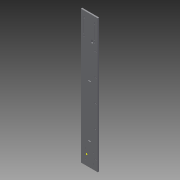
# Autodesk Inventor part: Tenda Wifi Buoy Mounting Plate
Saved by Autodesk Inventor 2015 (Build 190159000, 159)
## iProperties
Created: 2015-07-10
Part Number: Tenda Wifi Buoy Mounting Plate
Material: Generic
Document SubType Name: Modeling
Designer: Carey
Density: 1 g/cm^3
Appearance: Default
Author: Carey
Autodesk Inventor part; units mm, degrees
ref_plane "YZ Plane" through (0, 0, 0) normal (1, 0, 0) x (0, 1, 0)
ref_plane "XZ Plane" through (0, 0, 0) normal (0, 1, 0) x (-1, 0, 0)
ref_plane "XY Plane" through (0, 0, 0) normal (0, 0, 1) x (1, 0, 0)
sketch "Sketch1" plane through (0, 0, 0) normal (0, 0, 1) x (1, 0, 0)
  point P0 (0, 0)
sketch "Sketch2" plane through (0, 0, 0) normal (0, 0, 1) x (1, 0, 0)
  line L0 (-26.773, -46.7791) -> (49.427, -46.7791)
  line L1 (49.427, -46.7791) -> (49.427, 556.4709)
  line L2 (-26.773, 556.4709) -> (-26.773, -46.7791)
  line L3 (-13.7555, 533.9284) -> (-11.8505, 533.9284)
  line L4 (-11.8505, 533.9284) -> (-11.8505, 525.9909)
  line L5 (-11.8505, 525.9909) -> (-13.7555, 525.9909)
  line L6 (-13.7555, 525.9909) -> (-13.7555, 533.9284)
  line L7 (46.252, 424.6449) -> (44.347, 424.6449)
  line L8 (44.347, 424.6449) -> (44.347, 419.5649)
  line L9 (44.347, 419.5649) -> (46.252, 419.5649)
  line L10 (46.252, 419.5649) -> (46.252, 424.6449)
  line L11 (36.5111, 522.1809) -> (36.5111, 463.7609)
  line L12 (36.5111, 463.7609) -> (35.457, 463.7609)
  line L13 (35.457, 463.7609) -> (35.457, 522.1809)
  line L14 (35.457, 522.1809) -> (36.5111, 522.1809)
  line L15 (-13.7555, 522.1809) -> (-13.7555, 463.7609)
  line L16 (-13.7555, 463.7609) -> (-12.7014, 463.7609)
  line L17 (-12.7014, 463.7609) -> (-12.7014, 522.1809)
  line L18 (-12.7014, 522.1809) -> (-13.7555, 522.1809)
  line L19 (26.8845, 445.2941) -> (18.947, 445.2941)
  line L20 (18.947, 445.2941) -> (18.947, 457.9824)
  line L21 (18.947, 457.9824) -> (26.8845, 457.9824)
  line L22 (26.8845, 457.9824) -> (26.8845, 445.2941)
  line L23 (11.327, 54.8209) -> (17.677, 54.8209)
  line L24 (17.677, 54.8209) -> (17.677, 58.3769)
  line L25 (17.677, 58.3769) -> (4.977, 58.3769)
  line L26 (4.977, 58.3769) -> (4.977, 54.8209)
  line L27 (4.977, 54.8209) -> (11.327, 54.8209)
  line L28 (11.327, 293.7079) -> (17.677, 293.7079)
  line L29 (17.677, 293.7079) -> (17.677, 290.1519)
  line L30 (17.677, 290.1519) -> (4.977, 290.1519)
  line L31 (4.977, 290.1519) -> (4.977, 293.7079)
  line L32 (4.977, 293.7079) -> (11.327, 293.7079)
  line L33 (36.092, 424.6449) -> (37.997, 424.6449)
  line L34 (37.997, 424.6449) -> (37.997, 419.5649)
  line L35 (37.997, 419.5649) -> (36.092, 419.5649)
  line L36 (36.092, 419.5649) -> (36.092, 424.6449)
  line L37 (46.252, 323.0449) -> (44.347, 323.0449)
  line L38 (44.347, 323.0449) -> (44.347, 317.9649)
  line L39 (44.347, 317.9649) -> (46.252, 317.9649)
  line L40 (46.252, 317.9649) -> (46.252, 323.0449)
  line L41 (36.092, 323.0449) -> (37.997, 323.0449)
  line L42 (37.997, 323.0449) -> (37.997, 317.9649)
  line L43 (37.997, 317.9649) -> (36.092, 317.9649)
  line L44 (36.092, 317.9649) -> (36.092, 323.0449)
  line L45 (46.252, 221.4449) -> (44.347, 221.4449)
  line L46 (44.347, 221.4449) -> (44.347, 216.3649)
  line L47 (44.347, 216.3649) -> (46.252, 216.3649)
  line L48 (46.252, 216.3649) -> (46.252, 221.4449)
  line L49 (36.092, 221.4449) -> (37.997, 221.4449)
  line L50 (37.997, 221.4449) -> (37.997, 216.3649)
  line L51 (37.997, 216.3649) -> (36.092, 216.3649)
  line L52 (36.092, 216.3649) -> (36.092, 221.4449)
  line L53 (46.252, 0.1368) -> (44.347, 0.1368)
  line L54 (44.347, 0.1368) -> (44.347, -4.9432)
  line L55 (44.347, -4.9432) -> (46.252, -4.9432)
  line L56 (46.252, -4.9432) -> (46.252, 0.1368)
  line L57 (36.092, 0.1368) -> (37.997, 0.1368)
  line L58 (37.997, 0.1368) -> (37.997, -4.9432)
  line L59 (37.997, -4.9432) -> (36.092, -4.9432)
  line L60 (36.092, -4.9432) -> (36.092, 0.1368)
  line L61 (49.427, 556.4709) -> (-26.773, 556.4709)
  line L62 (46.252, 424.6449) -> (147.852, 424.6449) construction
  line L63 (46.252, 119.8449) -> (147.852, 119.8449) construction
  line L64 (46.252, 119.8449) -> (44.347, 119.8449)
  line L65 (44.347, 119.8449) -> (44.347, 114.7649)
  line L66 (44.347, 114.7649) -> (46.252, 114.7649)
  line L67 (46.252, 114.7649) -> (46.252, 119.8449)
  line L68 (36.092, 119.8449) -> (37.997, 119.8449)
  line L69 (36.092, 114.7649) -> (36.092, 119.8449)
  line L70 (37.997, 114.7649) -> (36.092, 114.7649)
  line L71 (37.997, 119.8449) -> (37.997, 114.7649)
  line L72 (36.5111, 533.9284) -> (34.6061, 533.9284)
  line L73 (34.6061, 533.9284) -> (34.6061, 525.9909)
  line L74 (34.6061, 525.9909) -> (36.5111, 525.9909)
  line L75 (36.5111, 525.9909) -> (36.5111, 533.9284)
  line L76 (-13.7555, 452.0134) -> (-11.8505, 452.0134)
  line L77 (-11.8505, 452.0134) -> (-11.8505, 459.9509)
  line L78 (-11.8505, 459.9509) -> (-13.7555, 459.9509)
  line L79 (-13.7555, 459.9509) -> (-13.7555, 452.0134)
  line L80 (34.6061, 459.9509) -> (36.5111, 459.9509)
  line L81 (34.6061, 452.0134) -> (34.6061, 459.9509)
  line L82 (36.5111, 459.9509) -> (36.5111, 452.0134)
  line L83 (36.5111, 452.0134) -> (34.6061, 452.0134)
  line L84 (29.4245, 23.0709) -> (31.3295, 23.0709)
  line L85 (31.3295, 23.0709) -> (31.3295, 15.1334)
  line L86 (29.4245, 15.1334) -> (29.4245, 23.0709)
  line L87 (31.3295, 15.1334) -> (29.4245, 15.1334)
  line L88 (-6.7705, 23.0709) -> (-8.6755, 23.0709)
  line L89 (-8.6755, 15.1334) -> (-6.7705, 15.1334)
  line L90 (-8.6755, 23.0709) -> (-8.6755, 15.1334)
  line L91 (-6.7705, 15.1334) -> (-6.7705, 23.0709)
  line L92 (30.3774, -19.8306) -> (32.2817, -19.7787)
  line L93 (32.4981, -27.7132) -> (30.5938, -27.7652)
  line L94 (32.2817, -19.7787) -> (32.4981, -27.7132)
  line L95 (30.5938, -27.7652) -> (30.3774, -19.8306)
  line L96 (-6.7705, -19.7916) -> (-8.6755, -19.7916)
  line L97 (-8.6755, -19.7916) -> (-8.6755, -27.7291)
  line L98 (-8.6755, -27.7291) -> (-6.7705, -27.7291)
  line L99 (-6.7705, -27.7291) -> (-6.7705, -19.7916)
  point P0 (30.377, 23.0709)
  point P1 (-7.723, 23.0709)
  point P2 (-7.723, 23.0709)
  point P3 (30.377, -19.7916)
  point P4 (-6.7705, -27.7291)
  point P5 (-7.723, -19.7916)
  point P6 (-7.723, -19.7916)
  dimension "d0" = 76.2
  dimension "d4" = 1.905
  dimension "d5" = 7.9375
  dimension "d8" = 58.42
  dimension "d13" = 7.9375
  dimension "d16" = 6.35
  dimension "d17" = 3.556
  dimension "d18" = 12.7
  constraints: 200 end point, 9 perpendicular, 6 horizontal, 4 parallel, 2 point on line, 1 collinear, 1 midpoint, 1 vertical
  measures "d0" distance of L0.start L0.end
  measures "d4" distance of L4.end L5.end
  measures "d5" distance of L3.end L4.end
  measures "d8" distance of L11.start L11.end
  measures "d13" distance of L19.start L19.end
  measures "d16" distance of L23.start L23.end
  measures "d17" distance of L23.end L24.end
  measures "d18" distance of L24.end L25.end
extrude "Extrusion3" add sketch "Sketch2" against normal blind 5.9944
body "Solid3"
